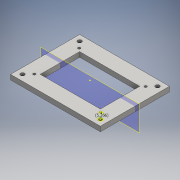
# Autodesk Inventor part: Joystickboard Holder
Saved by Autodesk Inventor 2016 SP2 (Build 200236200, 236)
## iProperties
Created: 2018-02-18
Part Number: Joystickboard Holder
Material: Generic
Document SubType Name: Modeling
Designer: Alexander
Density: 1 g/cm^3
Appearance: Default
Author: Alexander
Autodesk Inventor part; units mm, degrees
ref_plane "YZ Plane" through (0, 0, 0) normal (1, 0, 0) x (0, 1, 0)
ref_plane "XZ Plane" through (0, 0, 0) normal (0, 1, 0) x (-1, 0, 0)
ref_plane "XY Plane" through (0, 0, 0) normal (0, 0, 1) x (1, 0, 0)
sketch "Sketch1" plane through (0, 0, 0) normal (0, 0, 1) x (1, 0, 0)
  line L0 (-30.5, -20) -> (30.5, -20)
  line L1 (30.5, -20) -> (30.5, 20)
  line L2 (30.5, 20) -> (-30.5, 20)
  line L3 (-30.5, 20) -> (-30.5, -20)
  line L4 (-30.5, -20) -> (30.5, 20) construction
  line L5 (30.5, -20) -> (-30.5, 20) construction
  line L6 (-45.5, -35) -> (45.5, -35)
  line L7 (45.5, -35) -> (45.5, 35)
  line L8 (45.5, 35) -> (-45.5, 35)
  line L9 (-45.5, 35) -> (-45.5, -35)
  line L10 (-45.5, -35) -> (45.5, 35) construction
  line L11 (45.5, -35) -> (-45.5, 35) construction
  point P0 (0, 0)
  dimension "d0" = 61
  dimension "d1" = 40
  dimension "d2" = 15
  dimension "d3" = 15
  constraints: 24 end point, 4 midpoint, 4 parallel, 2 horizontal, 2 perpendicular
  measures "d0" distance of L1.end L2.end
  measures "d1" distance of L0.end L1.end
  measures "d2" distance between parallel lines of L8 L2
  measures "d3" distance between parallel lines of L7 L1
extrude "Rim" add sketch "Sketch1" along normal blind 5
sketch "Sketch2" plane through (0, 0, 5) normal (0, 0, 1) x (1, 0, 0)
  line L0 (-33.7, -22.765) -> (33.7, -22.765) construction
  line L1 (33.7, -22.765) -> (33.7, 22.765) construction
  line L2 (33.7, 22.765) -> (-33.7, 22.765) construction
  line L3 (-33.7, 22.765) -> (-33.7, -22.765) construction
  line L4 (-33.7, -22.765) -> (33.7, 22.765) construction
  line L5 (33.7, -22.765) -> (-33.7, 22.765) construction
  circle A0 centre (33.7, 22.765) radius 1.25
  line L6 (0, 22.765) -> (0, -22.765) construction
  line L7 (-30.5, -20) -> (-30.5, 20) projected
  line L8 (-30.5, 0) -> (33.7, 0) construction
  circle A1 centre (-33.7, 22.765) radius 1.25
  circle A2 centre (33.7, -22.765) radius 1.25
  circle A3 centre (-33.7, -22.765) radius 1.25
  point P0 (0, 0)
  dimension "d6" = 67.4
  dimension "d7" = 45.53
  dimension "d8" = 2.5
  constraints: 16 end point, 6 midpoint, 4 centre point, 3 symmetric about line, 2 parallel, 1 coincident, 1 horizontal, 1 perpendicular, 3 other
  measures "d6" distance of L1.end L2.end
  measures "d7" distance of L0.end L1.end
  measures "d8" diameter of A0
extrude "Pegs" cut sketch "Sketch2" against normal blind 3
sketch "Sketch4" plane through (0, 0, 0) normal (0, 0, -1) x (-1, 0, 0)
  circle A0 centre (-39.5, 29) radius 2 projected
  circle A1 centre (39.5, 29) radius 2 projected
  circle A2 centre (39.5, -29) radius 2 projected
  circle A3 centre (-39.5, -29) radius 2 projected
  point P0 (0, 0)
  constraints: 4 coincident
extrude "Bolt Holes" cut sketch "Sketch4" against normal up to next
sketch "For Construction" plane through (0, 0, 5) normal (0, 0, 1) x (1, 0, 0)
  circle A0 centre (33.7, -22.765) radius 1.25 projected
  circle A1 centre (39.5, -29) radius 2 projected
  point P0 (0, 0)
  point P1 (34.95, -22.765)
  point P2 (37.901, -27.7986)
  dimension "d19" = 5.2656
  constraints: 1 horizontal alignment, 3 other
ref_plane "Work Plane2" through (-30.5, 0, 0) normal (0, 1, 0) x (1, 0, 0)
sketch "Sketch13" plane through (0, 0, 0) normal (0, 0, -1) x (-1, 0, 0)
  circle A0 centre (-39.5, -29) radius 3
  circle A1 centre (-39.5, -29) radius 2 projected
  line L0 (45.5, -35) -> (-45.5, -35) projected
  line L1 (0, -35) -> (0, -20) construction
  line L2 (-30.5, -20) -> (30.5, -20) projected
  line L3 (-27.3467, 0) -> (-45.5, 0) construction
  line L4 (-45.5, -35) -> (-45.5, 35) projected
  line L5 (-45.5, -35) -> (-45.5, 35) projected
  circle A2 centre (-39.5, 29) radius 3
  circle A3 centre (39.5, -29) radius 3
  circle A4 centre (39.5, 29) radius 3
  point P0 (0, 0)
  dimension "d42" = 6
  constraints: 4 centre point, 4 end point, 4 midpoint, 3 symmetric about line, 2 coincident, 1 horizontal, 3 other
  measures "d42" diameter of A0
extrude "Bolt heads" cut sketch "Sketch13" against normal blind 3
body "Solid1"
